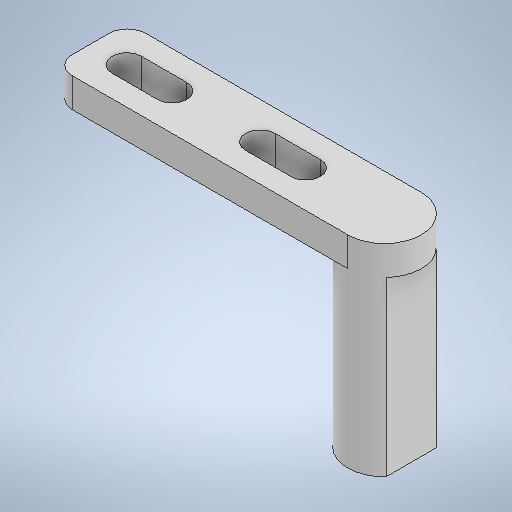
# Autodesk Inventor part: Sensor_Connect_Knob_Brake
Saved by Autodesk Inventor 2025 (Build 290162000, 162)
## iProperties
Created: 2024-11-19
Part Number: Sensor_Connect_Knob_Brake
Material: Generic
Document SubType Name: Modeling
Designer: phil
Density: 1 g/cm^3
Appearance: Default
Author: phil
Autodesk Inventor part; units mm, degrees
ref_plane "YZ Plane" through (0, 0, 0) normal (1, 0, 0) x (0, 1, 0)
ref_plane "XZ Plane" through (0, 0, 0) normal (0, 1, 0) x (-1, 0, 0)
ref_plane "XY Plane" through (0, 0, 0) normal (0, 0, 1) x (1, 0, 0)
sketch "Sketch1" plane through (0, 0, 0) normal (0, 1, 0) x (-1, 0, 0)
  arc A0 (-2.1359, -2.7727) -> (-2.1359, 2.7727) centre (0, 0) ccw
  line L0 (3.4641, 0.5) -> (-2.1359, 0.5)
  line L1 (-2.1359, 0.5) -> (-2.1359, -2.7727)
  line L2 (-2.1359, 0.5) -> (-2.1359, 2.7727)
  line L3 (-3.6359, 3.4322) -> (-3.6359, 0.5)
  line L4 (-3.6359, 0.5) -> (-3.6359, -3.4322)
  arc A1 (-3.6359, -3.4322) -> (-3.6359, 3.4322) centre (0, 0) ccw
  dimension "d0" = 7
  dimension "d1" = 5.6
  dimension "d2" = 3
  dimension "d3" = 1.5
  constraints: 10 end point, 5 point on circle, 2 centre point, 1 coincident, 1 horizontal, 1 perpendicular, 1 point on line, 2 other
  measures "d0" diameter of A0
  measures "d1" distance of L0.start L0.end
  measures "d2" distance edge to line of A0 L0
  measures "d3" radial gap between concentric circles of A0 A1
extrude "Extrusion1" add sketch "Sketch1" along normal blind 21
sketch "Sketch2" plane through (0, 21, 0) normal (0, 1, 0) x (1, 0, 0)
  line L0 (3.6359, -3.4322) -> (3.6359, 3.4322) projected
  arc A0 (3.6359, 3.4322) -> (3.6359, -3.4322) centre (0, 0) ccw projected
  line L1 (2.1359, 2.7727) -> (2.1359, -2.7727) projected
  arc A1 (2.1359, 2.7727) -> (2.1359, -2.7727) centre (0, 0) ccw projected
extrude "Extrusion2" add sketch "Sketch2" along normal blind 2.5 contours A0 L0 | L1 A1
sketch "Sketch4" plane through (0, 23.5, 0) normal (0, 1, 0) x (1, 0, 0)
  arc A0 (3.6359, 3.4322) -> (3.6359, -3.4322) centre (0, 0) ccw projected
  line L0 (3.6359, -3.4322) -> (3.6359, 3.4322) projected
  circle A1 centre (0, 0) radius 5
  line L1 (0, -5) -> (-37.5, -5)
  line L2 (-40, -2.5) -> (-40, 2.5)
  line L3 (-37.5, 5) -> (0, 5)
  arc A2 (-40, -2.5) -> (-37.5, -5) centre (-37.5, -2.5) ccw
  arc A3 (-37.5, 5) -> (-40, 2.5) centre (-37.5, 2.5) ccw
  line L4 (-35.0895, 0) -> (-28.9105, 0) construction
  line L5 (-35.0895, -2) -> (-28.9105, -2)
  line L6 (-28.9105, 2) -> (-35.0895, 2)
  arc A4 (-35.0895, 2) -> (-35.0895, -2) centre (-35.0895, 0) ccw
  arc A5 (-28.9105, -2) -> (-28.9105, 2) centre (-28.9105, 0) ccw
  line L7 (-22.9105, 5) -> (-22.9105, -5)
  line L8 (-10.7314, 0) -> (-16.9105, 0) construction
  line L9 (-10.7314, -2) -> (-16.9105, -2)
  line L10 (-16.9105, 2) -> (-10.7314, 2)
  arc A6 (-10.7314, -2) -> (-10.7314, 2) centre (-10.7314, 0) ccw
  arc A7 (-16.9105, 2) -> (-16.9105, -2) centre (-16.9105, 0) ccw
  point P0 (-40, -5)
  point P1 (-32, 0)
  point P2 (-40, 0)
  point P3 (-26.9105, 0)
  point P4 (-8.321, -2.5)
  point P5 (-8.321, 2.5)
  point P6 (-13.821, 0)
  point P7 (-18.9105, 0)
  point P8 (3.6359, -3.4322)
  point P9 (3.6359, 3.4322)
  dimension "d28" = 40
  dimension "d29" = 2.5
  dimension "d30" = 4
  dimension "d31" = 8
  dimension "d32" = 4
  dimension "d33" = 26.5464
  constraints: 24 end point, 15 point on circle, 12 tangent, 10 symmetric about line, 7 centre point, 4 point on line, 3 perpendicular, 2 horizontal, 2 midpoint, 1 coincident, 1 equal radius, 1 parallel, 2 other
  measures "d28" distance of L1.start point (-40, -5)
  measures "d29" radius of A2
  measures "d30" diameter of A5
  measures "d31" distance of point (-40, 0) point (-32, 0)
  measures "d32" distance from line of point (-26.91, 0) L7
  measures "d33" distance between parallel lines of L0 L7
extrude "Extrusion4" add sketch "Sketch4" along normal blind 4
body "Solid1"
